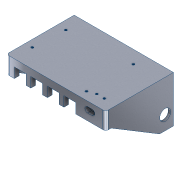
# Autodesk Inventor part: Base2
Saved by Autodesk Inventor 2020 (Build 240168000, 168)
## iProperties
Created: 2019-11-12
Part Number: Base2
Material: Generic
Document SubType Name: Modeling
Designer: Alex
Density: 1 g/cm^3
Appearance: Default
Author: Alex
Autodesk Inventor part; units mm, degrees
ref_plane "YZ Plane" through (0, 0, 0) normal (1, 0, 0) x (0, 1, 0)
ref_plane "XZ Plane" through (0, 0, 0) normal (0, 1, 0) x (-1, 0, 0)
ref_plane "XY Plane" through (0, 0, 0) normal (0, 0, 1) x (1, 0, 0)
ref_plane "Work Plane1" through (-47.911, 13.5701, 78.0288) normal (0, 0, 1) x (1, 0, 0)
sketch "Sketch1" plane through (0, 0, 0) normal (0, 0, 1) x (1, 0, 0)
  line L0 (-52.3875, -33.2867) -> (52.3875, -33.2867) projected
  arc A0 (52.3875, -33.2867) -> (57.15, -28.5242) centre (52.3875, -28.5242) ccw projected
  line L1 (57.15, -28.5242) -> (57.15, 33.2867) projected
  line L2 (57.15, 33.2867) -> (-57.15, 33.2867) projected
  line L3 (-57.15, 33.2867) -> (-57.15, -28.5242) projected
  arc A1 (-57.15, -28.5242) -> (-52.3875, -33.2867) centre (-52.3875, -28.5242) ccw projected
  circle A2 centre (52.3875, -28.5242) radius 1.524 construction
  circle A3 centre (52.3875, 28.5242) radius 1.524 construction
  circle A4 centre (-52.3875, 28.5242) radius 1.524 construction
  circle A5 centre (-52.3875, -28.5242) radius 1.524 construction
  circle A6 centre (52.3875, -28.5242) radius 1.1303
  circle A7 centre (52.3875, 28.5242) radius 1.1303
  circle A8 centre (-52.3875, 28.5242) radius 1.1303
  circle A9 centre (-52.3875, -28.5242) radius 1.1303
  line L4 (49.5554, 30.6197) -> (49.5554, -30.6197) projected
  line L5 (49.5554, -30.6197) -> (-49.5554, -30.6197) projected
  line L6 (-49.5554, -30.6197) -> (-49.5554, 30.6197) projected
  line L7 (-49.5554, 30.6197) -> (49.5554, 30.6197) projected
  line L8 (49.5554, 30.6197) -> (54.483, 30.6197)
  line L9 (54.483, 30.6197) -> (54.483, -30.6197)
  line L10 (54.483, -30.6197) -> (49.5554, -30.6197)
  line L11 (49.5554, -30.6197) -> (49.5554, 30.6197)
  line L12 (-49.5554, -30.6197) -> (-54.483, -30.6197)
  line L13 (-54.483, -30.6197) -> (-54.483, 30.6197)
  line L14 (-54.483, 30.6197) -> (-49.5554, 30.6197)
  line L15 (-49.5554, 30.6197) -> (-49.5554, -30.6197)
  point P0 (0, 0)
  dimension "d0" = 2.2606
  dimension "d16" = 2.667
  dimension "d17" = 2.667
  dimension "d18" = 2.667
  constraints: 16 end point, 4 centre point, 4 coincident, 4 parallel, 3 equal radius, 2 horizontal, 2 perpendicular
  measures "d0" diameter of A6
  measures "d16" distance between parallel lines of L2 L7
  measures "d17" distance between parallel lines of L1 L9
  measures "d18" distance between parallel lines of L3 L13
extrude "Extrusion1" add sketch "Sketch1" along normal up to surface (78.0288 mm away) contours A1 L3 L2 L1 A0 L0
sketch "Sketch2" plane through (-57.15, -28.5242, 0) normal (-1, 0, 0) x (0, 0, 1)
  line L0 (0, -4.7625) -> (78.0288, -4.7625) projected
  line L1 (78.0288, -4.7625) -> (78.0288, 42.0943)
  line L2 (78.0288, 42.0943) -> (71.6788, 42.0943)
  line L3 (71.6788, 42.0943) -> (15.875, 8.3693)
  line L4 (15.875, 8.3693) -> (0, 8.3693)
  line L5 (0, 8.3693) -> (0, -4.7625)
  point P0 (0, 28.5242)
  point P1 (-2.54, -1.5875)
  point P2 (-13.6652, 8.3693)
  dimension "d3" = 6.35
  dimension "d4" = 15.875
  constraints: 10 end point, 2 perpendicular, 1 horizontal alignment, 1 parallel, 1 vertical, 3 other
  measures "d3" distance of L1.end L2.end
  measures "d4" distance of L3.end L4.end
extrude "Extrusion2" cut sketch "Sketch2" against normal through all
sketch "Sketch3" plane through (-57.15, 33.2867, 78.0288) normal (0, 0, 1) x (1, 0, 0)
  line L0 (47.339, -8.2866) -> (60.547, -8.2866) projected
  line L1 (60.547, -8.2866) -> (60.547, -19.7166) projected
  line L2 (60.547, -19.7166) -> (47.339, -19.7166) construction
  line L3 (47.339, -19.7166) -> (47.339, -8.2866) projected
  line L4 (66.389, -8.2866) -> (79.597, -8.2866) projected
  line L5 (79.597, -8.2866) -> (79.597, -19.7166) projected
  line L6 (79.597, -19.7166) -> (66.389, -19.7166) construction
  line L7 (66.389, -19.7166) -> (66.389, -8.2866) projected
  line L8 (28.289, -8.2866) -> (41.497, -8.2866) projected
  line L9 (41.497, -8.2866) -> (41.497, -19.7166) projected
  line L10 (41.497, -19.7166) -> (28.289, -19.7166) construction
  line L11 (28.289, -19.7166) -> (28.289, -8.2866) projected
  line L12 (9.239, -8.2866) -> (22.447, -8.2866) projected
  line L13 (22.447, -8.2866) -> (22.447, -19.7166) projected
  line L14 (22.447, -19.7166) -> (9.239, -19.7166) construction
  line L15 (9.239, -19.7166) -> (9.239, -8.2866) projected
  line L16 (99.1941, -9.8795) -> (99.3441, -9.8795) construction
  arc A0 (99.3441, -9.8795) -> (99.8441, -9.3795) centre (99.3441, -9.3795) ccw construction
  line L17 (99.8441, -9.3795) -> (99.8441, -9.2545) construction
  line L18 (99.5441, -8.7545) -> (99.5441, -8.5623) construction
  arc A1 (99.8441, -8.5623) -> (99.6976, -8.2088) centre (99.3441, -8.5623) ccw construction
  line L19 (99.6976, -8.2088) -> (99.0648, -7.5759) construction
  arc A2 (99.0648, -7.5759) -> (98.7113, -7.4295) centre (98.7113, -7.9295) ccw construction
  line L20 (98.7113, -7.4295) -> (98.6941, -7.4295) construction
  line L21 (98.7113, -7.7295) -> (98.6941, -7.7295) construction
  arc A3 (98.8527, -7.7881) -> (98.7113, -7.7295) centre (98.7113, -7.9295) ccw construction
  line L22 (99.4855, -8.4209) -> (98.8527, -7.7881) construction
  arc A4 (99.5441, -8.5623) -> (99.4855, -8.4209) centre (99.3441, -8.5623) ccw construction
  line L23 (92.6441, -8.5623) -> (92.6441, -8.7545) construction
  arc A5 (92.7027, -8.4209) -> (92.6441, -8.5623) centre (92.8441, -8.5623) ccw construction
  line L24 (93.3355, -7.7881) -> (92.7027, -8.4209) construction
  arc A6 (93.4769, -7.7295) -> (93.3355, -7.7881) centre (93.4769, -7.9295) ccw construction
  line L25 (93.4941, -7.7295) -> (93.4769, -7.7295) construction
  line L26 (93.4941, -7.4295) -> (93.4769, -7.4295) construction
  arc A7 (93.4769, -7.4295) -> (93.1234, -7.5759) centre (93.4769, -7.9295) ccw construction
  line L27 (93.1234, -7.5759) -> (92.4905, -8.2088) construction
  arc A8 (92.4905, -8.2088) -> (92.3441, -8.5623) centre (92.8441, -8.5623) ccw construction
  line L28 (92.3441, -8.5623) -> (92.3441, -8.7545) construction
  line L29 (92.3441, -9.2545) -> (92.3441, -9.3795) construction
  arc A9 (92.3441, -9.3795) -> (92.8441, -9.8795) centre (92.8441, -9.3795) ccw construction
  line L30 (92.8441, -9.8795) -> (92.9941, -9.8795) construction
  line L31 (111.633, -2.667) -> (2.667, -2.667) projected
  line L32 (2.667, -19.7166) -> (9.239, -19.7166)
  line L33 (22.447, -19.7166) -> (28.289, -19.7166)
  line L34 (41.497, -19.7166) -> (47.339, -19.7166)
  line L35 (60.547, -19.7166) -> (66.389, -19.7166)
  line L36 (79.597, -19.7166) -> (111.633, -19.7166)
  line L37 (99.8441, -8.5623) -> (99.8441, -9.2545) construction
  line L38 (99.1941, -9.8795) -> (92.9941, -9.8795) construction
  line L39 (98.6941, -7.4295) -> (93.4769, -7.4295) construction
  line L40 (92.3441, -8.7545) -> (92.3441, -9.2545) construction
  line L41 (99.9711, -9.2545) -> (99.9711, -9.3795)
  arc A10 (99.3441, -10.0065) -> (99.9711, -9.3795) centre (99.3441, -9.3795) ccw
  line L42 (99.3441, -10.0065) -> (99.1941, -10.0065)
  line L43 (99.1941, -10.0065) -> (92.9941, -10.0065)
  line L44 (92.9941, -10.0065) -> (92.8441, -10.0065)
  arc A11 (92.2171, -9.3795) -> (92.8441, -10.0065) centre (92.8441, -9.3795) ccw
  line L45 (92.2171, -9.3795) -> (92.2171, -9.2545)
  line L46 (92.2171, -9.2545) -> (92.2171, -8.7545)
  line L47 (92.2171, -8.7545) -> (92.2171, -8.5623)
  arc A12 (92.4007, -8.119) -> (92.2171, -8.5623) centre (92.8441, -8.5623) ccw
  line L48 (92.4007, -8.119) -> (93.0336, -7.4861)
  arc A13 (93.4769, -7.3025) -> (93.0336, -7.4861) centre (93.4769, -7.9295) ccw
  line L49 (93.4769, -7.3025) -> (98.6941, -7.3025)
  line L50 (98.6941, -7.3025) -> (98.7113, -7.3025)
  arc A14 (99.1546, -7.4861) -> (98.7113, -7.3025) centre (98.7113, -7.9295) ccw
  line L51 (99.1546, -7.4861) -> (99.7875, -8.119)
  arc A15 (99.9711, -8.5623) -> (99.7875, -8.119) centre (99.3441, -8.5623) ccw
  line L52 (99.9711, -8.5623) -> (99.9711, -9.2545)
  line L53 (111.633, -19.7166) -> (111.633, -2.667) projected
  line L54 (2.667, -2.667) -> (2.667, -19.7166) projected
  point P0 (57.15, -33.2867)
  dimension "d7" = 0.127
  constraints: 42 end point, 12 point on circle, 6 centre point, 4 collinear, 4 perpendicular, 2 horizontal, 1 vertical, 17 other
  measures "d7" distance between parallel lines of L37 L52
ref_plane "Work Plane2" through (-52.102, 25.8572, 72.5424) normal (0, 0, 1) x (1, 0, 0)
extrude "Extrusion3" add sketch "Sketch3" against normal up to surface (5.4864 mm away)
thicken "Thicken1" operation cut thickness 0.127 both sides no extend neighbours no toward (1, 0, 0) faces at (22.447, 21.1901, 76.2) (12.109, 29.0745, 72.5424) (9.239, 17.3801, 76.2) (-9.811, 17.3801, 76.2) (-5.4083, 25.0001, 76.2) (13.6417, 25.0001, 74.3712) (3.397, 17.3801, 76.2) (-15.653, 21.1901, 76.2) (-24.4583, 25.0001, 74.3712) (-28.861, 17.3801, 76.2) (-43.5083, 25.0001, 74.3712) (-47.911, 17.3801, 76.2) (-34.703, 21.1901, 76.2)
sketch "Sketch4" plane through (-57.15, 33.2867, 78.0288) normal (0, 0, 1) x (1, 0, 0)
  line L0 (99.3441, -10.0065) -> (92.8441, -10.0065) construction
  line L1 (93.4769, -7.3025) -> (98.7113, -7.3025) construction
  line L2 (96.0941, -7.3025) -> (96.0941, -10.0065) construction
  line L3 (93.5541, -8.6545) -> (98.6341, -8.6545) construction
  line L4 (93.5541, -11.8295) -> (98.6341, -11.8295)
  line L5 (98.6341, -5.4795) -> (93.5541, -5.4795)
  arc A0 (93.5541, -5.4795) -> (93.5541, -11.8295) centre (93.5541, -8.6545) ccw
  arc A1 (98.6341, -11.8295) -> (98.6341, -5.4795) centre (98.6341, -8.6545) ccw
  point P0 (57.15, -33.2867)
  point P1 (96.0941, -8.6545)
  dimension "d13" = 5.08
  dimension "d82" = 6.35
  constraints: 10 end point, 4 midpoint, 4 point on circle, 4 tangent, 2 centre point, 1 horizontal, 1 parallel
  measures "d13" distance of L3.start L3.end
  measures "d82" distance between parallel lines of L5 L4
extrude "Extrusion4" cut sketch "Sketch4" against normal blind 4.5594
sketch "Sketch5" plane through (-54.483, 30.6197, 0) normal (0, -1, 0) x (1, 0, 0)
  circle A0 centre (80.4225, 14.8209) radius 1.651 construction
  circle A1 centre (97.8723, 65.5574) radius 1.524 construction
  circle A2 centre (88.9823, 65.5574) radius 1.524 construction
  circle A3 centre (80.4225, 68.7324) radius 1.651 construction
  circle A4 centre (5.3655, 56.2229) radius 1.905 construction
  circle A5 centre (7.334, 19.5834) radius 1.651 construction
  circle A6 centre (80.4225, 14.8209) radius 3.81
  circle A7 centre (97.8723, 65.5574) radius 3.81
  circle A8 centre (88.9823, 65.5574) radius 3.81
  circle A9 centre (80.4225, 68.7324) radius 3.81
  circle A10 centre (5.3655, 56.2229) radius 3.81
  circle A11 centre (7.334, 19.5834) radius 3.81
  circle A12 centre (80.4225, 14.8209) radius 1.1303
  circle A13 centre (7.334, 19.5834) radius 1.1303
  circle A14 centre (5.3655, 56.2229) radius 1.1303
  circle A15 centre (80.4225, 68.7324) radius 1.1303
  circle A16 centre (88.9823, 65.5574) radius 1.1303
  circle A17 centre (97.8723, 65.5574) radius 1.1303
  point P0 (54.483, 0)
  dimension "d19" = 7.62
  dimension "d20" = 2.2606
  constraints: 12 centre point, 12 coincident, 10 equal radius
  measures "d19" diameter of A6
  measures "d20" diameter of A12
ref_plane "Work Plane3" through (-52.102, 27.4447, 11.5824) normal (0, 1, 0) x (0, 0, 1)
extrude "Extrusion5" add sketch "Sketch5" along normal up to surface (3.175 mm away)
sketch "Sketch6" plane through (-57.15, 33.2867, 0) normal (-1, 0, 0) x (0, 0, 1)
  arc A0 (31.7313, -23.2525) -> (32.4313, -23.9525) centre (32.4313, -23.2525) ccw construction
  line L0 (38.7313, -23.9525) -> (32.4313, -23.9525) construction
  arc A1 (38.7313, -23.9525) -> (39.4313, -23.2525) centre (38.7313, -23.2525) ccw construction
  line L1 (39.4313, -22.4559) -> (39.4313, -23.2525) construction
  arc A2 (39.4313, -22.4559) -> (39.2286, -21.9633) centre (38.7313, -22.4559) ccw construction
  line L2 (39.0031, -21.7356) -> (39.2286, -21.9633) construction
  arc A3 (38.9163, -21.5245) -> (39.0031, -21.7356) centre (39.2163, -21.5245) ccw construction
  line L3 (38.9163, -20.7525) -> (38.9163, -21.5245) construction
  arc A4 (38.9163, -20.7525) -> (38.2163, -20.0525) centre (38.2163, -20.7525) ccw construction
  line L4 (32.9463, -20.0525) -> (38.2163, -20.0525) construction
  arc A5 (32.9463, -20.0525) -> (32.2463, -20.7525) centre (32.9463, -20.7525) ccw construction
  line L5 (32.2463, -21.5245) -> (32.2463, -20.7525) construction
  arc A6 (32.1594, -21.7356) -> (32.2463, -21.5245) centre (31.9463, -21.5245) ccw construction
  line L6 (31.9339, -21.9633) -> (32.1594, -21.7356) construction
  arc A7 (31.9339, -21.9633) -> (31.7313, -22.4559) centre (32.4313, -22.4559) ccw construction
  line L7 (31.7313, -23.2525) -> (31.7313, -22.4559) construction
  line L8 (32.337, -21.9116) -> (32.1115, -22.1393) construction
  arc A8 (32.337, -21.9116) -> (32.4963, -21.5245) centre (31.9463, -21.5245) ccw construction
  line L9 (32.4963, -20.7525) -> (32.4963, -21.5245) construction
  arc A9 (32.9463, -20.3025) -> (32.4963, -20.7525) centre (32.9463, -20.7525) ccw construction
  line L10 (38.2163, -20.3025) -> (32.9463, -20.3025) construction
  arc A10 (38.6663, -20.7525) -> (38.2163, -20.3025) centre (38.2163, -20.7525) ccw construction
  line L11 (38.6663, -21.5245) -> (38.6663, -20.7525) construction
  arc A11 (38.6663, -21.5245) -> (38.8255, -21.9116) centre (39.2163, -21.5245) ccw construction
  line L12 (39.051, -22.1393) -> (38.8255, -21.9116) construction
  arc A12 (39.1813, -22.4559) -> (39.051, -22.1393) centre (38.7313, -22.4559) ccw construction
  line L13 (39.1813, -23.2525) -> (39.1813, -22.4559) construction
  arc A13 (38.7313, -23.7025) -> (39.1813, -23.2525) centre (38.7313, -23.2525) ccw construction
  line L14 (32.4313, -23.7025) -> (38.7313, -23.7025) construction
  arc A14 (31.9813, -23.2525) -> (32.4313, -23.7025) centre (32.4313, -23.2525) ccw construction
  line L15 (31.9813, -22.4559) -> (31.9813, -23.2525) construction
  arc A15 (32.1115, -22.1393) -> (31.9813, -22.4559) centre (32.4313, -22.4559) ccw construction
  arc A16 (38.7313, -24.0915) -> (39.5703, -23.2525) centre (38.7313, -23.2525) ccw
  line L16 (38.7313, -24.0915) -> (32.4313, -24.0915)
  arc A17 (31.5923, -23.2525) -> (32.4313, -24.0915) centre (32.4313, -23.2525) ccw
  line L17 (31.5923, -23.2525) -> (31.5923, -22.4559)
  arc A18 (31.8351, -21.8655) -> (31.5923, -22.4559) centre (32.4313, -22.4559) ccw
  line L18 (31.8351, -21.8655) -> (32.0607, -21.6378)
  arc A19 (32.0607, -21.6378) -> (32.1073, -21.5245) centre (31.9463, -21.5245) ccw
  line L19 (32.1073, -21.5245) -> (32.1073, -20.7525)
  arc A20 (32.9463, -19.9135) -> (32.1073, -20.7525) centre (32.9463, -20.7525) ccw
  line L20 (32.9463, -19.9135) -> (38.2163, -19.9135)
  arc A21 (39.0553, -20.7525) -> (38.2163, -19.9135) centre (38.2163, -20.7525) ccw
  line L21 (39.0553, -20.7525) -> (39.0553, -21.5245)
  arc A22 (39.0553, -21.5245) -> (39.1019, -21.6378) centre (39.2163, -21.5245) ccw
  line L22 (39.1019, -21.6378) -> (39.3274, -21.8655)
  arc A23 (39.5703, -22.4559) -> (39.3274, -21.8655) centre (38.7313, -22.4559) ccw
  line L23 (39.5703, -22.4559) -> (39.5703, -23.2525)
  point P0 (0, -33.2867)
  constraints: 16 end point, 16 point on circle, 8 centre point, 15 other
extrude "Extrusion6" cut sketch "Sketch6" against normal up to next
sketch "Sketch7" plane through (-57.15, -20.1549, 0) normal (0, -1, 0) x (1, 0, 0)
  line L0 (2.667, 71.6788) -> (2.667, 15.875) construction
  line L1 (0, 31.5923) -> (2.667, 31.5923)
  line L2 (2.667, 31.5923) -> (2.667, 39.5703)
  line L3 (2.667, 39.5703) -> (0, 39.5703)
  line L4 (0, 39.5703) -> (0, 31.5923) construction
  line L5 (2.667, 39.5703) -> (0.5, 39.5703)
  line L6 (0.5, 39.5703) -> (0.5, 31.5923)
  line L7 (0.5, 31.5923) -> (2.667, 31.5923)
  line L8 (2.667, 31.5923) -> (2.667, 39.5703)
  point P0 (57.15, 0)
  dimension "d31" = 0.5
  constraints: 16 end point, 4 parallel, 2 horizontal, 2 perpendicular, 2 point on line, 1 coincident
  measures "d31" distance between parallel lines of L4 L6
extrude "Extrusion7" cut sketch "Sketch7" against normal up to surface (33.5281 mm away)
sketch "Sketch8" plane through (-56.65, -10.6562, 31.5923) normal (1, 0, 0) x (0, 0, -1)
  line L0 (0, 0) -> (-7.978, 4.8215) projected
  line L1 (0, 0) -> (0, 20.6904) projected
  line L2 (-7.978, 4.8215) -> (-7.978, 20.6904) projected
  line L3 (-7.978, 24.0294) -> (0, 24.0294) projected
  line L4 (0, 12.0914) -> (-7.978, 12.0914)
  line L5 (-46.4365, 24.2263) -> (-28.2755, 24.2263) construction
  line L6 (-46.4365, 35.6563) -> (-42.436, 35.6563) construction
  point P0 (31.5923, 10.6562)
  dimension "d34" = 11.43
  dimension "d35" = 11.938
  constraints: 2 end point, 2 point on line, 1 perpendicular
  measures "d34" distance between parallel lines of L6 L5
  measures "d35" distance between parallel lines of L3 L4
extrude "Extrusion8" add sketch "Sketch8" along normal up to surface (2.167 mm away)
sketch "Sketch9" plane through (0, 0, 0) normal (0, 0, -1) x (-1, 0, 0)
  circle A0 centre (52.3875, 28.5242) radius 3.175 construction
  circle A1 centre (-52.3875, 28.5242) radius 3.175 construction
  line L0 (-54.483, 30.6197) -> (-49.2125, 30.6197)
  line L1 (-49.2125, 30.6197) -> (-49.2125, 25.3492)
  line L2 (-49.2125, 25.3492) -> (-54.483, 25.3492)
  line L3 (-54.483, 25.3492) -> (-54.483, 30.6197)
  line L4 (54.483, 30.6197) -> (49.2125, 30.6197)
  line L5 (49.2125, 30.6197) -> (49.2125, 25.3492)
  line L6 (49.2125, 25.3492) -> (54.483, 25.3492)
  line L7 (54.483, 25.3492) -> (54.483, 30.6197)
  circle A2 centre (-52.3875, 28.5242) radius 1.1303
  circle A3 centre (52.3875, 28.5242) radius 1.1303
  point P0 (0, 0)
  dimension "d38" = 2.2606
  constraints: 16 end point, 4 parallel, 4 tangent, 2 centre point, 2 coincident, 2 horizontal, 2 perpendicular, 1 equal radius
  measures "d38" diameter of A2
extrude "Extrusion9" add sketch "Sketch9" against normal blind 6.35
fillet "Fillet1" radius 3.175 2 edges at (57.15, 23.4284, 78.0288) (-57.15, 23.4284, 78.0288)
sketch "Sketch10" plane through (54.483, -20.1549, 0) normal (-1, 0, 0) x (0, 0, 1)
  line L0 (11.43, 3.175) -> (3.175, 3.175)
  line L1 (3.175, 3.175) -> (3.175, 5.715)
  line L2 (3.175, 5.715) -> (11.43, 5.715)
  line L3 (11.43, 5.715) -> (11.43, 3.175)
  line L4 (68.5038, 36.9) -> (60.2488, 36.9)
  line L5 (60.2488, 36.9) -> (60.2488, 39.44)
  line L6 (60.2488, 39.44) -> (68.5038, 39.44)
  line L7 (68.5038, 39.44) -> (68.5038, 36.9)
  line L8 (74.8538, 33.725) -> (71.6788, 33.725) projected
  line L9 (15.875, 0) -> (0, 0) projected
  line L10 (0, 0) -> (0, 53.4416) projected
  point P0 (0, 20.1549)
  dimension "d43" = 8.255
  dimension "d44" = 2.54
  dimension "d45" = 3.175
  dimension "d46" = 3.175
  dimension "d47" = 3.175
  dimension "d48" = 3.175
  constraints: 16 end point, 6 parallel, 2 horizontal, 2 perpendicular
  measures "d43" distance of L1.end L2.end
  measures "d44" distance of L0.end L1.end
  measures "d45" distance between parallel lines of L8 L4
  measures "d46" distance between parallel lines of L9 L0
  measures "d47" distance between parallel lines of L10 L1
  measures "d48" distance from line of L8.end L7
extrude "Extrusion10" cut sketch "Sketch10" against normal blind 1.27
mirror "Mirror1" about plane through (0, 0, 0) normal (1, 0, 0) of "Extrusion10"
chamfer "Chamfer1" distance 1.27 angle 45 6 edges at (-50.959, 27.4447, 19.5834) (-52.9275, 27.4447, 56.2229) (22.1295, 27.4447, 68.7324) (30.6893, 27.4447, 65.5574) (39.5793, 27.4447, 65.5574) (22.1295, 27.4447, 14.8209)
chamfer "Chamfer2" distance 0.3175 angle 45 8 edges at (24.8092, 27.4447, 14.8209) (-48.2793, 27.4447, 19.5834) (-50.2478, 27.4447, 56.2229) (24.8092, 27.4447, 68.7324) (33.369, 27.4447, 65.5574) (42.259, 27.4447, 65.5574) (53.5178, 28.5242, 0) (-51.2572, 28.5242, 0)
ref_plane "Work Plane4" through (43.3893, 27.4447, 65.5574) normal (-1, 0, 0) x (0, 0, 1)
sketch "Sketch11" plane through (43.3893, 27.4447, 65.5574) normal (0, -1, 0) x (1, 0, 0)
  line L0 (-92.6018, -59.2074) -> (-92.6018, -65.5574) construction
  line L1 (-92.6018, -65.5574) -> (5.8232, -65.5574) construction
  line L2 (5.8232, -65.5574) -> (5.8232, -59.2074) construction
  line L3 (5.8232, -59.2074) -> (11.0937, -59.2074) construction
  line L4 (11.0937, 7.112) -> (11.0937, -59.2074) construction
  line L5 (11.0937, 7.112) -> (-97.8723, 7.112) construction
  line L6 (-97.8723, 7.112) -> (-97.8723, -59.2074) construction
  line L7 (-97.8723, -59.2074) -> (-92.6018, -59.2074) construction
  circle A0 centre (-17.4498, -50.7365) radius 3.81 construction
  circle A1 centre (-8.89, 0) radius 3.81 construction
  circle A2 centre (-92.5068, -9.3345) radius 3.81 construction
  circle A3 centre (-90.5383, -45.974) radius 3.81 construction
  circle A4 centre (0, 0) radius 3.81 construction
  circle A5 centre (-17.4498, 3.175) radius 3.81 construction
  circle A6 centre (0, 0) radius 1.1303
  circle A7 centre (-8.89, 0) radius 1.1303
  circle A8 centre (-17.4498, 3.175) radius 1.1303
  circle A9 centre (-17.4498, -50.7365) radius 1.1303
  circle A10 centre (-90.5383, -45.974) radius 1.1303
  circle A11 centre (-92.5068, -9.3345) radius 1.1303
  point P0 (-43.3893, -65.5574)
extrude "Extrusion11" cut sketch "Sketch11" against normal through all
sketch "Sketch12" plane through (43.3893, 27.4447, 65.5574) normal (-1, 0, 0) x (0, 0, 1)
  line L0 (1.1303, 0.3175) -> (-1.1303, 0.3175) construction
  line L1 (-1.4478, 0) -> (1.4478, 0) construction
  line L2 (-1.1303, 3.175) -> (1.1303, 3.175) construction
  line L3 (-1.1303, 5.842) -> (1.1303, 5.842) construction
  line L4 (0, 0) -> (0, 5.842)
  line L5 (-1.1303, -0.4762) -> (-1.1303, 0)
  line L6 (-1.1303, 0) -> (-1.4053, -0.1587)
  line L7 (-1.4053, -0.1587) -> (-1.4053, -0.3175)
  line L8 (-1.4053, -0.3175) -> (-1.1303, -0.4762)
  point P0 (-65.5574, -27.4447)
  dimension "d53" = 60
  dimension "d54" = 0.4763
  dimension "d55" = 0.1588
  dimension "d56" = 6.3182
  constraints: 10 end point, 2 midpoint, 1 equal length, 1 parallel, 1 point on line, 1 vertical, 1 vertical alignment
  measures "d53" angle of L6 L8
  measures "d54" distance of L5.start L5.end
  measures "d55" distance of L6.end L7.end
  measures "d56" distance from line of L3 L5.start
coil "Coil1" sketch "Sketch12" operation cut axis through (43.3893, 27.4447, 65.5574) along (0, 1, 0) pitch 0.635 turns 9.95 hand right
pattern_sketch "Sketch Driven Pattern1" of "Coil1" from (43.3893, 27.4447, 65.5574) copies at (34.4993, 27.4447, 65.5574) at (25.9395, 27.4447, 68.7324) at (25.9395, 27.4447, 14.8209) at (-49.1175, 27.4447, 56.2229) at (-47.149, 27.4447, 19.5834)
sketch "Sketch13" plane through (0, 0, 0) normal (0, 0, -1) x (-1, 0, 0)
  circle A0 centre (52.3875, 28.5242) radius 1.524 construction
  circle A1 centre (-52.3875, 28.5242) radius 1.524 construction
  point P0 (0, 0)
  constraints: 2 coincident
ref_plane "Work Plane5" through (-52.3875, 28.5242, 0) normal (0, 1, 0) x (1, 0, 0)
sketch "Sketch14" plane through (-52.3875, 28.5242, 0) normal (0, 1, 0) x (1, 0, 0)
  line L0 (-1.1303, -0.3175) -> (1.1303, -0.3175) construction
  line L1 (1.4478, 0) -> (-1.4478, 0) construction
  line L2 (1.1303, -6.35) -> (-1.1303, -6.35) construction
  line L3 (0, 0) -> (0, -6.35)
  line L4 (1.1303, 0.4763) -> (1.1303, 0)
  line L5 (1.1303, 0) -> (1.4053, 0.1588)
  line L6 (1.4053, 0.1588) -> (1.4053, 0.3175)
  line L7 (1.4053, 0.3175) -> (1.1303, 0.4763)
  point P0 (52.3875, 0)
  dimension "d65" = 60
  dimension "d66" = 0.4763
  dimension "d67" = 0.1588
  dimension "d68" = 6.8262
  constraints: 10 end point, 2 midpoint, 1 equal length, 1 parallel, 1 point on line, 1 vertical, 1 vertical alignment
  measures "d65" angle of L5 L7
  measures "d66" distance of L4.start L4.end
  measures "d67" distance of L5.end L6.end
  measures "d68" distance from line of L2 L4.start
coil "Coil2" sketch "Sketch14" operation cut axis through (-52.3875, 28.5242, 0) along (0, 0, 1) pitch 0.635 turns 10.75 hand right
pattern_sketch "Sketch Driven Pattern2" of "Coil2" from (-52.3875, 28.5242, 0) copies at (52.3875, 28.5242, 0)
sketch "Sketch15" plane through (57.15, -20.1549, 0) normal (1, 0, 0) x (0, 0, -1)
  circle A0 centre (-9.525, 15.875) radius 6.35
  line L0 (0, 0) -> (0, 53.4416) projected
  line L1 (-15.875, 0) -> (0, 0) projected
  point P0 (0, 20.1549)
  dimension "d77" = 12.7
  dimension "d78" = 9.525
  dimension "d79" = 15.875
  constraints: 1 centre point
  measures "d77" diameter of A0
  measures "d78" distance from line of L0 A0.centre
  measures "d79" distance from line of L1 A0.centre
extrude "Extrusion12" cut sketch "Sketch15" against normal up to next
equation "\"d17\" = d16"
equation "\"d18\" = d16"
equation "\"d46\" = d45"
equation "\"d47\" = d46"
equation "\"d48\" = d45"
equation "\"d55\" = 0.333333 * d54"
equation "\"d58\" = d56"
equation "\"d67\" = 0.333333 * d66"
equation "\"d70\" = d68"
body "Solid1"
